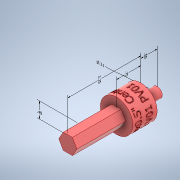
# Autodesk Inventor part: 1x8mmx1_5-inchHexShaft
Saved by Autodesk Inventor 2022.2 (Build 262287000, 287)
## iProperties
Created: 2020-11-16
Part Number: 1x8mmx1_5-inchHexShaft
Material: PC/ABS Plastic
Document SubType Name: Modeling
Designer: robst
Density: 0.357273 g/cm^3
Appearance: Smooth - Red
Author: robst
Autodesk Inventor part; units mm, degrees
ref_plane "XZ Plane" through (0, 0, 0) normal (0, 1, 0) x (-1, 0, 0)
ref_plane "XY Plane" through (0, 0, 0) normal (0, 0, 1) x (1, 0, 0)
sketch "Sketch1" plane through (0, 0, 0) normal (0, 0, 1) x (1, 0, 0)
  line L0 (7.3323, 0) -> (3.6662, -6.35)
  line L1 (3.6662, -6.35) -> (-3.6662, -6.35)
  line L2 (-3.6662, -6.35) -> (-7.3323, 0)
  line L3 (-7.3323, 0) -> (-3.6662, 6.35)
  line L4 (-3.6662, 6.35) -> (3.6662, 6.35)
  line L5 (3.6662, 6.35) -> (7.3323, 0)
  point P0 (0, 0)
  point P1 (0, 0)
  dimension "d0" = 12.7
  constraints: 12 end point, 1 coincident, 1 horizontal, 13 other
  measures "d0" distance between parallel lines of L1 L4
extrude "Hex Portion" add sketch "Sketch1" along normal mid plane 38.1
sketch "Sketch2" plane through (0, 0, -19.05) normal (0, 0, -1) x (-1, 0, 0)
  circle A0 centre (0, 0) radius 12.7
  dimension "d3" = 25.4
  constraints: 1 centre point, 1 coincident
  measures "d3" diameter of A0
extrude "Extrusion2" add sketch "Sketch2" along normal blind 19.05
thicken "Reduce Size of Hex Shaft" operation add thickness 0.1905 both sides no extend neighbours yes toward (-0.8660254, -0.5, 0) faces at (6.1103, 2.1167, -6.35) (-1.2221, 6.35, 6.35) (4.8882, -4.2333, -6.35) (-1.2221, -6.35, -6.35) (-4.8882, -4.2333, 6.35) (-6.1103, 2.1167, 6.35)
sketch "Sketch3" plane through (0, 0, -38.1) normal (0, 0, -1) x (-1, 0, 0)
  circle A0 centre (0, 0) radius 4
  dimension "d14" = 8
  constraints: 1 centre point, 1 coincident
  measures "d14" diameter of A0
extrude "Extrusion3" add sketch "Sketch3" along normal blind 12.7
ref_plane "Work Plane1" through (12.7, 0, -19.05) normal (1, 0, 0) x (0, 1, 0)
sketch "Sketch4" plane through (12.7, 0, -19.05) normal (1, 0, 0) x (0, 1, 0)
  line L0 (-12.7, 0) -> (12.7, 0) projected
  line L1 (-12.7, -19.05) -> (12.7, -19.05) projected
  line L2 (-12.7, 0) -> (-12.7, -19.05) construction
  line L3 (-12.7, -9.525) -> (12.7, -9.525) construction
  line L4 (12.7, 0) -> (12.7, -19.05) construction
  line L5 (-28.8024, -6.985) -> (-31.2807, -6.985)
  line L6 (-31.2807, -6.985) -> (-31.2807, -6.4663)
  line L7 (-31.2807, -6.4663) -> (-30.3586, -6.4663)
  line L8 (-30.3586, -6.4663) -> (-30.3586, -3.0618)
  line L9 (-30.3586, -3.0618) -> (-31.2807, -3.0618)
  line L10 (-31.2807, -3.0618) -> (-31.2807, -2.5966)
  spline S0 degree 2 poles (-31.2807, -2.5966) (-30.7579, -2.5966) (-30.2639, -2.3002) (-30.2309, -1.8885) knots 0 0 0 1 2 2 2
  line L11 (-30.2309, -1.8885) -> (-29.704, -1.8885)
  line L12 (-29.704, -1.8885) -> (-29.704, -6.4663)
  line L13 (-29.704, -6.4663) -> (-28.8024, -6.4663)
  line L14 (-28.8024, -6.4663) -> (-28.8024, -6.985)
  line L15 (-27.1064, -1.6786) -> (-27.2546, -3.6546)
  line L16 (-27.2546, -3.6546) -> (-27.7033, -3.6546)
  line L17 (-27.7033, -3.6546) -> (-27.8515, -1.6786)
  line L18 (-27.8515, -1.6786) -> (-27.1064, -1.6786)
  line L19 (-25.822, -1.6786) -> (-25.9702, -3.6546)
  line L20 (-25.9702, -3.6546) -> (-26.4189, -3.6546)
  line L21 (-26.4189, -3.6546) -> (-26.5671, -1.6786)
  line L22 (-26.5671, -1.6786) -> (-25.822, -1.6786)
  line L23 (-22.0099, -6.985) -> (-22.7962, -6.985)
  line L24 (-22.7962, -6.985) -> (-23.7224, -5.5524)
  line L25 (-23.7224, -5.5524) -> (-24.6734, -6.985)
  line L26 (-24.6734, -6.985) -> (-25.4021, -6.985)
  line L27 (-25.4021, -6.985) -> (-24.0806, -5.0954)
  line L28 (-24.0806, -5.0954) -> (-25.3897, -3.1729)
  line L29 (-25.3897, -3.1729) -> (-24.6034, -3.1729)
  line L30 (-24.6034, -3.1729) -> (-23.6813, -4.5932)
  line L31 (-23.6813, -4.5932) -> (-22.7386, -3.1729)
  line L32 (-22.7386, -3.1729) -> (-22.0099, -3.1729)
  line L33 (-22.0099, -3.1729) -> (-23.3231, -5.0543)
  line L34 (-23.3231, -5.0543) -> (-22.0099, -6.985)
  spline S1 degree 2 poles (-20.0709, -7.1003) (-20.4497, -7.1003) (-21.0713, -6.8738) (-21.2895, -6.6639) knots 0 0 0 1 2 2 2
  spline S2 degree 2 poles (-21.2895, -6.6639) (-21.5035, -6.4581) (-21.7259, -5.8982) (-21.7259, -5.5812) knots 0 0 0 1 2 2 2
  spline S3 degree 2 poles (-21.7259, -5.5812) (-21.7259, -5.1695) (-21.2854, -4.4779) (-20.8655, -4.2721) knots 0 0 0 1 2 2 2
  line L35 (-20.8655, -4.2721) -> (-20.8655, -4.2515)
  spline S4 degree 2 poles (-20.8655, -4.2515) (-21.2401, -4.0333) (-21.6024, -3.5146) (-21.6024, -3.1277) knots 0 0 0 1 2 2 2
  spline S5 degree 2 poles (-21.6024, -3.1277) (-21.6024, -2.5554) (-20.7378, -1.7897) (-20.0709, -1.7897) knots 0 0 0 1 2 2 2
  spline S6 degree 2 poles (-20.0709, -1.7897) (-19.3793, -1.7897) (-18.5436, -2.5143) (-18.5436, -3.0824) knots 0 0 0 1 2 2 2
  spline S7 degree 2 poles (-18.5436, -3.0824) (-18.5436, -3.4241) (-18.943, -4.091) (-19.3176, -4.2803) knots 0 0 0 1 2 2 2
  line L36 (-19.3176, -4.2803) -> (-19.3176, -4.3009)
  spline S8 degree 2 poles (-19.3176, -4.3009) (-18.873, -4.5068) (-18.416, -5.0996) (-18.416, -5.5689) knots 0 0 0 1 2 2 2
  spline S9 degree 2 poles (-18.416, -5.5689) (-18.416, -6.2193) (-19.3629, -7.1003) (-20.0709, -7.1003) knots 0 0 0 1 2 2 2
  spline S10 degree 2 poles (-19.1159, -5.6347) (-19.1159, -5.3219) (-19.3629, -4.9514) (-19.7128, -4.762) knots 0 0 0 1 2 2 2
  spline S11 degree 2 poles (-19.7128, -4.762) (-19.8281, -4.6961) (-20.215, -4.5438) (-20.4579, -4.445) knots 0 0 0 1 2 2 2
  spline S12 degree 2 poles (-20.4579, -4.445) (-20.7378, -4.6303) (-21.0384, -5.1819) (-21.0384, -5.5318) knots 0 0 0 1 2 2 2
  spline S13 degree 2 poles (-21.0384, -5.5318) (-21.0384, -5.9929) (-20.4826, -6.5939) (-20.0627, -6.5939) knots 0 0 0 1 2 2 2
  spline S14 degree 2 poles (-20.0627, -6.5939) (-19.6346, -6.5939) (-19.1159, -6.0793) (-19.1159, -5.6347) knots 0 0 0 1 2 2 2
  spline S15 degree 2 poles (-19.2106, -3.0906) (-19.2106, -2.7489) (-19.6675, -2.292) (-20.0751, -2.292) knots 0 0 0 1 2 2 2
  spline S16 degree 2 poles (-20.0751, -2.292) (-20.4456, -2.292) (-20.919, -2.6995) (-20.919, -3.0494) knots 0 0 0 1 2 2 2
  spline S17 degree 2 poles (-20.919, -3.0494) (-20.919, -3.3006) (-20.6761, -3.6505) (-20.4332, -3.7904) knots 0 0 0 1 2 2 2
  spline S18 degree 2 poles (-20.4332, -3.7904) (-20.3303, -3.8481) (-19.8939, -4.0498) (-19.7169, -4.1074) knots 0 0 0 1 2 2 2
  spline S19 degree 2 poles (-19.7169, -4.1074) (-19.4205, -3.881) (-19.2106, -3.3994) (-19.2106, -3.0906) knots 0 0 0 1 2 2 2
  line L37 (-13.3772, -6.985) -> (-13.3772, -4.7785)
  spline S20 degree 2 poles (-13.3772, -4.7785) (-13.3772, -4.515) (-13.4184, -4.0663) (-13.4842, -3.9428) knots 0 0 0 1 2 2 2
  spline S21 degree 2 poles (-13.4842, -3.9428) (-13.5501, -3.8069) (-13.8012, -3.6752) (-14.0194, -3.6752) knots 0 0 0 1 2 2 2
  spline S22 degree 2 poles (-14.0194, -3.6752) (-14.217, -3.6752) (-14.6698, -3.9181) (-14.9086, -4.1486) knots 0 0 0 1 2 2 2
  spline S23 degree 2 poles (-14.9086, -4.1486) (-14.9045, -4.2062) (-14.8963, -4.3668) (-14.8963, -4.4738) knots 0 0 0 1 2 2 2
  line L38 (-14.8963, -4.4738) -> (-14.8963, -6.985)
  line L39 (-14.8963, -6.985) -> (-15.5385, -6.985)
  line L40 (-15.5385, -6.985) -> (-15.5385, -4.7785)
  spline S24 degree 2 poles (-15.5385, -4.7785) (-15.5385, -4.515) (-15.5796, -4.0663) (-15.6455, -3.9428) knots 0 0 0 1 2 2 2
  spline S25 degree 2 poles (-15.6455, -3.9428) (-15.7114, -3.8069) (-15.9625, -3.6752) (-16.1807, -3.6752) knots 0 0 0 1 2 2 2
  spline S26 degree 2 poles (-16.1807, -3.6752) (-16.3865, -3.6752) (-16.8435, -3.9345) (-17.0575, -4.1362) knots 0 0 0 1 2 2 2
  line L41 (-17.0575, -4.1362) -> (-17.0575, -6.985)
  line L42 (-17.0575, -6.985) -> (-17.6997, -6.985)
  line L43 (-17.6997, -6.985) -> (-17.6997, -3.1729)
  line L44 (-17.6997, -3.1729) -> (-17.0575, -3.1729)
  line L45 (-17.0575, -3.1729) -> (-17.0575, -3.5928)
  spline S27 degree 2 poles (-17.0575, -3.5928) (-16.8064, -3.3417) (-16.3124, -3.0659) (-16.016, -3.0659) knots 0 0 0 1 2 2 2
  spline S28 degree 2 poles (-16.016, -3.0659) (-15.6784, -3.0659) (-15.1556, -3.3747) (-15.0198, -3.7246) knots 0 0 0 1 2 2 2
  spline S29 degree 2 poles (-15.0198, -3.7246) (-14.7275, -3.3994) (-14.1758, -3.0659) (-13.8547, -3.0659) knots 0 0 0 1 2 2 2
  spline S30 degree 2 poles (-13.8547, -3.0659) (-13.6077, -3.0659) (-13.2043, -3.2182) (-13.0561, -3.3911) knots 0 0 0 1 2 2 2
  spline S31 degree 2 poles (-13.0561, -3.3911) (-12.9038, -3.564) (-12.735, -4.0827) (-12.735, -4.4738) knots 0 0 0 1 2 2 2
  line L46 (-12.735, -4.4738) -> (-12.735, -6.985)
  line L47 (-12.735, -6.985) -> (-13.3772, -6.985)
  line L48 (-7.5109, -6.985) -> (-7.5109, -4.7785)
  spline S32 degree 2 poles (-7.5109, -4.7785) (-7.5109, -4.515) (-7.5521, -4.0663) (-7.6179, -3.9428) knots 0 0 0 1 2 2 2
  spline S33 degree 2 poles (-7.6179, -3.9428) (-7.6838, -3.8069) (-7.9349, -3.6752) (-8.1531, -3.6752) knots 0 0 0 1 2 2 2
  spline S34 degree 2 poles (-8.1531, -3.6752) (-8.3507, -3.6752) (-8.8035, -3.9181) (-9.0423, -4.1486) knots 0 0 0 1 2 2 2
  spline S35 degree 2 poles (-9.0423, -4.1486) (-9.0382, -4.2062) (-9.03, -4.3668) (-9.03, -4.4738) knots 0 0 0 1 2 2 2
  line L49 (-9.03, -4.4738) -> (-9.03, -6.985)
  line L50 (-9.03, -6.985) -> (-9.6722, -6.985)
  line L51 (-9.6722, -6.985) -> (-9.6722, -4.7785)
  spline S36 degree 2 poles (-9.6722, -4.7785) (-9.6722, -4.515) (-9.7133, -4.0663) (-9.7792, -3.9428) knots 0 0 0 1 2 2 2
  spline S37 degree 2 poles (-9.7792, -3.9428) (-9.8451, -3.8069) (-10.0962, -3.6752) (-10.3144, -3.6752) knots 0 0 0 1 2 2 2
  spline S38 degree 2 poles (-10.3144, -3.6752) (-10.5202, -3.6752) (-10.9772, -3.9345) (-11.1912, -4.1362) knots 0 0 0 1 2 2 2
  line L52 (-11.1912, -4.1362) -> (-11.1912, -6.985)
  line L53 (-11.1912, -6.985) -> (-11.8334, -6.985)
  line L54 (-11.8334, -6.985) -> (-11.8334, -3.1729)
  line L55 (-11.8334, -3.1729) -> (-11.1912, -3.1729)
  line L56 (-11.1912, -3.1729) -> (-11.1912, -3.5928)
  spline S39 degree 2 poles (-11.1912, -3.5928) (-10.9401, -3.3417) (-10.4461, -3.0659) (-10.1497, -3.0659) knots 0 0 0 1 2 2 2
  spline S40 degree 2 poles (-10.1497, -3.0659) (-9.8121, -3.0659) (-9.2893, -3.3747) (-9.1535, -3.7246) knots 0 0 0 1 2 2 2
  spline S41 degree 2 poles (-9.1535, -3.7246) (-8.8612, -3.3994) (-8.3095, -3.0659) (-7.9884, -3.0659) knots 0 0 0 1 2 2 2
  spline S42 degree 2 poles (-7.9884, -3.0659) (-7.7414, -3.0659) (-7.338, -3.2182) (-7.1898, -3.3911) knots 0 0 0 1 2 2 2
  spline S43 degree 2 poles (-7.1898, -3.3911) (-7.0375, -3.564) (-6.8687, -4.0827) (-6.8687, -4.4738) knots 0 0 0 1 2 2 2
  line L57 (-6.8687, -4.4738) -> (-6.8687, -6.985)
  line L58 (-6.8687, -6.985) -> (-7.5109, -6.985)
  line L59 (-3.0072, -6.985) -> (-3.7935, -6.985)
  line L60 (-3.7935, -6.985) -> (-4.7198, -5.5524)
  line L61 (-4.7198, -5.5524) -> (-5.6707, -6.985)
  line L62 (-5.6707, -6.985) -> (-6.3994, -6.985)
  line L63 (-6.3994, -6.985) -> (-5.0779, -5.0954)
  line L64 (-5.0779, -5.0954) -> (-6.3871, -3.1729)
  line L65 (-6.3871, -3.1729) -> (-5.6008, -3.1729)
  line L66 (-5.6008, -3.1729) -> (-4.6786, -4.5932)
  line L67 (-4.6786, -4.5932) -> (-3.7359, -3.1729)
  line L68 (-3.7359, -3.1729) -> (-3.0072, -3.1729)
  line L69 (-3.0072, -3.1729) -> (-4.3205, -5.0543)
  line L70 (-4.3205, -5.0543) -> (-3.0072, -6.985)
  spline S44 degree 2 poles (0.5578, -4.445) (0.5578, -5.8117) (-0.2367, -7.092) (-1.0642, -7.092) knots 0 0 0 1 2 2 2
  spline S45 degree 2 poles (-1.0642, -7.092) (-1.904, -7.092) (-2.6903, -5.787) (-2.6903, -4.4491) knots 0 0 0 1 2 2 2
  spline S46 degree 2 poles (-2.6903, -4.4491) (-2.6903, -3.0741) (-1.8957, -1.8021) (-1.0642, -1.8021) knots 0 0 0 1 2 2 2
  spline S47 degree 2 poles (-1.0642, -1.8021) (-0.2285, -1.8021) (0.5578, -3.1194) (0.5578, -4.445) knots 0 0 0 1 2 2 2
  spline S48 degree 2 poles (-0.3149, -5.9929) (-0.2161, -5.7418) (-0.1338, -4.9678) (-0.1338, -4.445) knots 0 0 0 1 2 2 2
  spline S49 degree 2 poles (-0.1338, -4.445) (-0.1338, -3.9222) (-0.2161, -3.1524) (-0.319, -2.893) knots 0 0 0 1 2 2 2
  spline S50 degree 2 poles (-0.319, -2.893) (-0.422, -2.6337) (-0.7801, -2.3661) (-1.0642, -2.3661) knots 0 0 0 1 2 2 2
  spline S51 degree 2 poles (-1.0642, -2.3661) (-1.3482, -2.3661) (-1.7146, -2.6337) (-1.8216, -2.9012) knots 0 0 0 1 2 2 2
  spline S52 degree 2 poles (-1.8216, -2.9012) (-1.9246, -3.1606) (-1.9987, -3.951) (-1.9987, -4.4491) knots 0 0 0 1 2 2 2
  spline S53 degree 2 poles (-1.9987, -4.4491) (-1.9987, -4.9843) (-1.9328, -5.7006) (-1.8258, -5.9805) knots 0 0 0 1 2 2 2
  spline S54 degree 2 poles (-1.8258, -5.9805) (-1.727, -6.244) (-1.3606, -6.528) (-1.0642, -6.528) knots 0 0 0 1 2 2 2
  spline S55 degree 2 poles (-1.0642, -6.528) (-0.7842, -6.528) (-0.4178, -6.2605) (-0.3149, -5.9929) knots 0 0 0 1 2 2 2
  line L71 (2.2992, -6.985) -> (1.4841, -6.985)
  line L72 (1.4841, -6.985) -> (1.4841, -6.0135)
  line L73 (1.4841, -6.0135) -> (2.2992, -6.0135)
  line L74 (2.2992, -6.0135) -> (2.2992, -6.985)
  spline S56 degree 2 poles (6.4035, -5.3713) (6.4035, -5.7376) (6.1689, -6.3634) (5.9548, -6.5939) knots 0 0 0 1 2 2 2
  spline S57 degree 2 poles (5.9548, -6.5939) (5.7407, -6.8244) (5.1026, -7.092) (4.7074, -7.092) knots 0 0 0 1 2 2 2
  spline S58 degree 2 poles (4.7074, -7.092) (4.3452, -7.092) (3.6371, -6.9315) (3.3777, -6.8039) knots 0 0 0 1 2 2 2
  line L75 (3.3777, -6.8039) -> (3.3777, -6.0834)
  line L76 (3.3777, -6.0834) -> (3.4271, -6.0834)
  spline S59 degree 2 poles (3.4271, -6.0834) (3.5054, -6.1411) (3.7976, -6.2893) (3.9747, -6.3551) knots 0 0 0 1 2 2 2
  spline S60 degree 2 poles (3.9747, -6.3551) (4.1764, -6.4251) (4.5098, -6.5033) (4.7198, -6.5033) knots 0 0 0 1 2 2 2
  spline S61 degree 2 poles (4.7198, -6.5033) (4.9256, -6.5033) (5.3126, -6.3551) (5.4526, -6.1946) knots 0 0 0 1 2 2 2
  spline S62 degree 2 poles (5.4526, -6.1946) (5.5802, -6.0423) (5.7119, -5.6388) (5.7119, -5.3671) knots 0 0 0 1 2 2 2
  spline S63 degree 2 poles (5.7119, -5.3671) (5.7119, -5.0954) (5.5637, -4.7496) (5.4237, -4.6344) knots 0 0 0 1 2 2 2
  spline S64 degree 2 poles (5.4237, -4.6344) (5.2797, -4.5068) (4.8515, -4.3997) (4.5922, -4.3997) knots 0 0 0 1 2 2 2
  spline S65 degree 2 poles (4.5922, -4.3997) (4.3122, -4.3997) (3.7565, -4.4862) (3.5877, -4.5232) knots 0 0 0 1 2 2 2
  line L77 (3.5877, -4.5232) -> (3.5877, -1.905)
  line L78 (3.5877, -1.905) -> (6.3747, -1.905)
  line L79 (6.3747, -1.905) -> (6.3747, -2.5019)
  line L80 (6.3747, -2.5019) -> (4.2423, -2.5019)
  line L81 (4.2423, -2.5019) -> (4.2423, -3.8563)
  spline S66 degree 2 poles (4.2423, -3.8563) (4.3658, -3.8398) (4.6045, -3.8275) (4.7033, -3.8275) knots 0 0 0 1 2 2 2
  spline S67 degree 2 poles (4.7033, -3.8275) (5.0944, -3.8275) (5.6337, -3.9551) (5.8807, -4.1445) knots 0 0 0 1 2 2 2
  spline S68 degree 2 poles (5.8807, -4.1445) (6.1318, -4.3338) (6.4035, -4.9102) (6.4035, -5.3713) knots 0 0 0 1 2 2 2
  line L82 (7.8979, -1.6786) -> (7.7497, -3.6546)
  line L83 (7.7497, -3.6546) -> (7.301, -3.6546)
  line L84 (7.301, -3.6546) -> (7.1528, -1.6786)
  line L85 (7.1528, -1.6786) -> (7.8979, -1.6786)
  line L86 (9.1823, -1.6786) -> (9.0341, -3.6546)
  line L87 (9.0341, -3.6546) -> (8.5854, -3.6546)
  line L88 (8.5854, -3.6546) -> (8.4372, -1.6786)
  line L89 (8.4372, -1.6786) -> (9.1823, -1.6786)
  spline S69 degree 2 poles (14.2499, -7.0756) (13.7559, -7.0756) (12.9202, -6.7421) (12.6156, -6.4087) knots 0 0 0 1 2 2 2
  spline S70 degree 2 poles (12.6156, -6.4087) (12.311, -6.0793) (11.9775, -5.0913) (11.9775, -4.4491) knots 0 0 0 1 2 2 2
  spline S71 degree 2 poles (11.9775, -4.4491) (11.9775, -3.811) (12.3027, -2.8642) (12.6115, -2.5143) knots 0 0 0 1 2 2 2
  spline S72 degree 2 poles (12.6115, -2.5143) (12.9161, -2.1726) (13.7477, -1.8144) (14.2623, -1.8144) knots 0 0 0 1 2 2 2
  spline S73 degree 2 poles (14.2623, -1.8144) (14.5175, -1.8144) (14.9662, -1.8885) (15.1556, -1.9462) knots 0 0 0 1 2 2 2
  spline S74 degree 2 poles (15.1556, -1.9462) (15.3203, -1.9997) (15.662, -2.152) (15.8307, -2.2426) knots 0 0 0 1 2 2 2
  line L90 (15.8307, -2.2426) -> (15.8307, -3.0577)
  line L91 (15.8307, -3.0577) -> (15.7772, -3.0577)
  spline S75 degree 2 poles (15.7772, -3.0577) (15.6867, -2.9753) (15.4067, -2.7448) (15.205, -2.6337) knots 0 0 0 1 2 2 2
  spline S76 degree 2 poles (15.205, -2.6337) (15.0115, -2.5266) (14.5546, -2.3908) (14.2582, -2.3908) knots 0 0 0 1 2 2 2
  spline S77 degree 2 poles (14.2582, -2.3908) (13.9329, -2.3908) (13.3525, -2.6584) (13.1343, -2.9136) knots 0 0 0 1 2 2 2
  spline S78 degree 2 poles (13.1343, -2.9136) (12.9202, -3.1729) (12.6815, -3.9592) (12.6815, -4.4491) knots 0 0 0 1 2 2 2
  spline S79 degree 2 poles (12.6815, -4.4491) (12.6815, -4.9719) (12.9326, -5.7253) (13.1508, -5.9846) knots 0 0 0 1 2 2 2
  spline S80 degree 2 poles (13.1508, -5.9846) (13.3648, -6.2358) (13.9371, -6.491) (14.2582, -6.491) knots 0 0 0 1 2 2 2
  spline S81 degree 2 poles (14.2582, -6.491) (14.5505, -6.491) (15.0486, -6.3469) (15.2421, -6.2399) knots 0 0 0 1 2 2 2
  spline S82 degree 2 poles (15.2421, -6.2399) (15.4273, -6.1328) (15.7031, -5.9105) (15.7813, -5.8323) knots 0 0 0 1 2 2 2
  line L92 (15.7813, -5.8323) -> (15.8307, -5.8323)
  line L93 (15.8307, -5.8323) -> (15.8307, -6.6392)
  spline S83 degree 2 poles (15.8307, -6.6392) (15.662, -6.7174) (15.3656, -6.8615) (15.1556, -6.9274) knots 0 0 0 1 2 2 2
  spline S84 degree 2 poles (15.1556, -6.9274) (14.9333, -7.0015) (14.5546, -7.0756) (14.2499, -7.0756) knots 0 0 0 1 2 2 2
  spline S85 degree 2 poles (18.0661, -7.0715) (17.1522, -7.0715) (16.1477, -6.0464) (16.1477, -5.0996) knots 0 0 0 1 2 2 2
  spline S86 degree 2 poles (16.1477, -5.0996) (16.1477, -4.1692) (17.1234, -3.0659) (17.9097, -3.0659) knots 0 0 0 1 2 2 2
  spline S87 degree 2 poles (17.9097, -3.0659) (18.2637, -3.0659) (18.8112, -3.2717) (19.0129, -3.4899) knots 0 0 0 1 2 2 2
  spline S88 degree 2 poles (19.0129, -3.4899) (19.2188, -3.7081) (19.437, -4.338) (19.437, -4.7949) knots 0 0 0 1 2 2 2
  line L94 (19.437, -4.7949) -> (19.437, -5.1448)
  line L95 (19.437, -5.1448) -> (16.7982, -5.1448)
  spline S89 degree 2 poles (16.7982, -5.1448) (16.7982, -5.8076) (17.4651, -6.5116) (18.0579, -6.5116) knots 0 0 0 1 2 2 2
  spline S90 degree 2 poles (18.0579, -6.5116) (18.2678, -6.5116) (18.6754, -6.4169) (18.84, -6.3428) knots 0 0 0 1 2 2 2
  spline S91 degree 2 poles (18.84, -6.3428) (19.0129, -6.2605) (19.2517, -6.1164) (19.3299, -6.0505) knots 0 0 0 1 2 2 2
  line L96 (19.3299, -6.0505) -> (19.367, -6.0505)
  line L97 (19.367, -6.0505) -> (19.367, -6.7503)
  spline S92 degree 2 poles (19.367, -6.7503) (19.2558, -6.7956) (18.9183, -6.9274) (18.7865, -6.9644) knots 0 0 0 1 2 2 2
  spline S93 degree 2 poles (18.7865, -6.9644) (18.6013, -7.0179) (18.2966, -7.0715) (18.0661, -7.0715) knots 0 0 0 1 2 2 2
  spline S94 degree 2 poles (18.8112, -4.655) (18.803, -4.3956) (18.696, -4.0169) (18.593, -3.8892) knots 0 0 0 1 2 2 2
  spline S95 degree 2 poles (18.593, -3.8892) (18.4819, -3.7452) (18.132, -3.5928) (17.8726, -3.5928) knots 0 0 0 1 2 2 2
  spline S96 degree 2 poles (17.8726, -3.5928) (17.6174, -3.5928) (17.2592, -3.7452) (17.111, -3.8934) knots 0 0 0 1 2 2 2
  spline S97 degree 2 poles (17.111, -3.8934) (16.967, -4.0457) (16.8188, -4.4121) (16.7982, -4.655) knots 0 0 0 1 2 2 2
  line L98 (16.7982, -4.655) -> (18.8112, -4.655)
  line L99 (23.0802, -6.985) -> (22.438, -6.985)
  line L100 (22.438, -6.985) -> (22.438, -4.8114)
  spline S98 degree 2 poles (22.438, -4.8114) (22.438, -4.5479) (22.3886, -4.0951) (22.3145, -3.9592) knots 0 0 0 1 2 2 2
  spline S99 degree 2 poles (22.3145, -3.9592) (22.2363, -3.8151) (21.9564, -3.6752) (21.7176, -3.6752) knots 0 0 0 1 2 2 2
  spline S100 degree 2 poles (21.7176, -3.6752) (21.4788, -3.6752) (20.9725, -3.9304) (20.7296, -4.1362) knots 0 0 0 1 2 2 2
  line L101 (20.7296, -4.1362) -> (20.7296, -6.985)
  line L102 (20.7296, -6.985) -> (20.0874, -6.985)
  line L103 (20.0874, -6.985) -> (20.0874, -3.1729)
  line L104 (20.0874, -3.1729) -> (20.7296, -3.1729)
  line L105 (20.7296, -3.1729) -> (20.7296, -3.597)
  spline S101 degree 2 poles (20.7296, -3.597) (21.0178, -3.3376) (21.5735, -3.0659) (21.8864, -3.0659) knots 0 0 0 1 2 2 2
  spline S102 degree 2 poles (21.8864, -3.0659) (22.4463, -3.0659) (23.0802, -3.8069) (23.0802, -4.5109) knots 0 0 0 1 2 2 2
  line L106 (23.0802, -4.5109) -> (23.0802, -6.985)
  spline S103 degree 2 poles (25.1345, -7.0591) (24.6117, -7.0591) (24.023, -6.4622) (24.023, -5.8159) knots 0 0 0 1 2 2 2
  line L107 (24.023, -5.8159) -> (24.023, -3.704)
  line L108 (24.023, -3.704) -> (23.5907, -3.704)
  line L109 (23.5907, -3.704) -> (23.5907, -3.1729)
  line L110 (23.5907, -3.1729) -> (24.023, -3.1729)
  line L111 (24.023, -3.1729) -> (24.023, -2.0779)
  line L112 (24.023, -2.0779) -> (24.6652, -2.0779)
  line L113 (24.6652, -2.0779) -> (24.6652, -3.1729)
  line L114 (24.6652, -3.1729) -> (25.8467, -3.1729)
  line L115 (25.8467, -3.1729) -> (25.8467, -3.704)
  line L116 (25.8467, -3.704) -> (24.6652, -3.704)
  line L117 (24.6652, -3.704) -> (24.6652, -5.5195)
  spline S104 degree 2 poles (24.6652, -5.5195) (24.6652, -5.8076) (24.6858, -6.1246) (24.7557, -6.2605) knots 0 0 0 1 2 2 2
  spline S105 degree 2 poles (24.7557, -6.2605) (24.8134, -6.3798) (25.0727, -6.4992) (25.295, -6.4992) knots 0 0 0 1 2 2 2
  spline S106 degree 2 poles (25.295, -6.4992) (25.4515, -6.4992) (25.7437, -6.4045) (25.8096, -6.3757) knots 0 0 0 1 2 2 2
  line L118 (25.8096, -6.3757) -> (25.8467, -6.3757)
  line L119 (25.8467, -6.3757) -> (25.8467, -6.9521)
  spline S107 degree 2 poles (25.8467, -6.9521) (25.6655, -7.0015) (25.295, -7.0591) (25.1345, -7.0591) knots 0 0 0 1 2 2 2
  spline S108 degree 2 poles (27.975, -7.0715) (27.0611, -7.0715) (26.0566, -6.0464) (26.0566, -5.0996) knots 0 0 0 1 2 2 2
  spline S109 degree 2 poles (26.0566, -5.0996) (26.0566, -4.1692) (27.0323, -3.0659) (27.8186, -3.0659) knots 0 0 0 1 2 2 2
  spline S110 degree 2 poles (27.8186, -3.0659) (28.1726, -3.0659) (28.7201, -3.2717) (28.9218, -3.4899) knots 0 0 0 1 2 2 2
  spline S111 degree 2 poles (28.9218, -3.4899) (29.1277, -3.7081) (29.3459, -4.338) (29.3459, -4.7949) knots 0 0 0 1 2 2 2
  line L120 (29.3459, -4.7949) -> (29.3459, -5.1448)
  line L121 (29.3459, -5.1448) -> (26.7071, -5.1448)
  spline S112 degree 2 poles (26.7071, -5.1448) (26.7071, -5.8076) (27.374, -6.5116) (27.9668, -6.5116) knots 0 0 0 1 2 2 2
  spline S113 degree 2 poles (27.9668, -6.5116) (28.1767, -6.5116) (28.5843, -6.4169) (28.7489, -6.3428) knots 0 0 0 1 2 2 2
  spline S114 degree 2 poles (28.7489, -6.3428) (28.9218, -6.2605) (29.1606, -6.1164) (29.2388, -6.0505) knots 0 0 0 1 2 2 2
  line L122 (29.2388, -6.0505) -> (29.2759, -6.0505)
  line L123 (29.2759, -6.0505) -> (29.2759, -6.7503)
  spline S115 degree 2 poles (29.2759, -6.7503) (29.1647, -6.7956) (28.8271, -6.9274) (28.6954, -6.9644) knots 0 0 0 1 2 2 2
  spline S116 degree 2 poles (28.6954, -6.9644) (28.5102, -7.0179) (28.2055, -7.0715) (27.975, -7.0715) knots 0 0 0 1 2 2 2
  spline S117 degree 2 poles (28.7201, -4.655) (28.7119, -4.3956) (28.6048, -4.0169) (28.5019, -3.8892) knots 0 0 0 1 2 2 2
  spline S118 degree 2 poles (28.5019, -3.8892) (28.3908, -3.7452) (28.0409, -3.5928) (27.7815, -3.5928) knots 0 0 0 1 2 2 2
  spline S119 degree 2 poles (27.7815, -3.5928) (27.5263, -3.5928) (27.1681, -3.7452) (27.0199, -3.8934) knots 0 0 0 1 2 2 2
  spline S120 degree 2 poles (27.0199, -3.8934) (26.8758, -4.0457) (26.7276, -4.4121) (26.7071, -4.655) knots 0 0 0 1 2 2 2
  line L124 (26.7071, -4.655) -> (28.7201, -4.655)
  line L125 (32.0176, -3.8604) -> (31.9847, -3.8604)
  spline S121 degree 2 poles (31.9847, -3.8604) (31.9106, -3.8398) (31.75, -3.8316) (31.6388, -3.8316) knots 0 0 0 1 2 2 2
  spline S122 degree 2 poles (31.6388, -3.8316) (31.3795, -3.8316) (30.869, -4.058) (30.6385, -4.2803) knots 0 0 0 1 2 2 2
  line L126 (30.6385, -4.2803) -> (30.6385, -6.985)
  line L127 (30.6385, -6.985) -> (29.9963, -6.985)
  line L128 (29.9963, -6.985) -> (29.9963, -3.1729)
  line L129 (29.9963, -3.1729) -> (30.6385, -3.1729)
  line L130 (30.6385, -3.1729) -> (30.6385, -3.741)
  spline S123 degree 2 poles (30.6385, -3.741) (30.9884, -3.4282) (31.5112, -3.1729) (31.7582, -3.1729) knots 0 0 0 1 2 2 2
  spline S124 degree 2 poles (31.7582, -3.1729) (31.857, -3.1729) (31.9558, -3.1812) (32.0176, -3.1935) knots 0 0 0 1 2 2 2
  line L131 (32.0176, -3.1935) -> (32.0176, -3.8604)
  spline S125 degree 2 poles (-21.979, -15.6168) (-22.5307, -15.6168) (-23.3046, -15.3863) (-23.6463, -15.2216) knots 0 0 0 1 2 2 2
  line L132 (-23.6463, -15.2216) -> (-23.6463, -14.3735)
  line L133 (-23.6463, -14.3735) -> (-23.5969, -14.3735)
  spline S126 degree 2 poles (-23.5969, -14.3735) (-23.2634, -14.6864) (-22.4195, -15.0322) (-22.0284, -15.0322) knots 0 0 0 1 2 2 2
  spline S127 degree 2 poles (-22.0284, -15.0322) (-21.4686, -15.0322) (-20.8963, -14.567) (-20.8963, -14.1842) knots 0 0 0 1 2 2 2
  spline S128 degree 2 poles (-20.8963, -14.1842) (-20.8963, -13.8795) (-21.1969, -13.5008) (-21.5221, -13.4061) knots 0 0 0 1 2 2 2
  spline S129 degree 2 poles (-21.5221, -13.4061) (-21.7567, -13.3403) (-22.1478, -13.2497) (-22.4401, -13.1756) knots 0 0 0 1 2 2 2
  spline S130 degree 2 poles (-22.4401, -13.1756) (-22.7036, -13.1056) (-23.1194, -12.8957) (-23.2799, -12.7269) knots 0 0 0 1 2 2 2
  spline S131 degree 2 poles (-23.2799, -12.7269) (-23.4363, -12.5581) (-23.6092, -12.1053) (-23.6092, -11.8088) knots 0 0 0 1 2 2 2
  spline S132 degree 2 poles (-23.6092, -11.8088) (-23.6092, -11.1913) (-22.6459, -10.3557) (-21.9008, -10.3557) knots 0 0 0 1 2 2 2
  spline S133 degree 2 poles (-21.9008, -10.3557) (-21.4727, -10.3557) (-20.7152, -10.5244) (-20.39, -10.685) knots 0 0 0 1 2 2 2
  line L134 (-20.39, -10.685) -> (-20.39, -11.4919)
  line L135 (-20.39, -11.4919) -> (-20.4394, -11.4919)
  spline S134 degree 2 poles (-20.4394, -11.4919) (-20.6823, -11.2696) (-21.4397, -10.9402) (-21.8555, -10.9402) knots 0 0 0 1 2 2 2
  spline S135 degree 2 poles (-21.8555, -10.9402) (-22.3248, -10.9402) (-22.9053, -11.3807) (-22.9053, -11.7389) knots 0 0 0 1 2 2 2
  spline S136 degree 2 poles (-22.9053, -11.7389) (-22.9053, -12.06) (-22.5636, -12.4428) (-22.2425, -12.5293) knots 0 0 0 1 2 2 2
  spline S137 degree 2 poles (-22.2425, -12.5293) (-22.0284, -12.5869) (-21.4068, -12.7351) (-21.201, -12.7969) knots 0 0 0 1 2 2 2
  spline S138 degree 2 poles (-21.201, -12.7969) (-20.6782, -12.9574) (-20.1924, -13.6037) (-20.1924, -14.0771) knots 0 0 0 1 2 2 2
  spline S139 degree 2 poles (-20.1924, -14.0771) (-20.1924, -14.3777) (-20.4353, -14.954) (-20.6535, -15.1557) knots 0 0 0 1 2 2 2
  spline S140 degree 2 poles (-20.6535, -15.1557) (-20.8963, -15.378) (-21.5138, -15.6168) (-21.979, -15.6168) knots 0 0 0 1 2 2 2
  line L136 (-16.5615, -15.5262) -> (-17.2037, -15.5262)
  line L137 (-17.2037, -15.5262) -> (-17.2037, -13.3526)
  spline S141 degree 2 poles (-17.2037, -13.3526) (-17.2037, -13.0891) (-17.2531, -12.6363) (-17.3272, -12.5005) knots 0 0 0 1 2 2 2
  spline S142 degree 2 poles (-17.3272, -12.5005) (-17.4054, -12.3564) (-17.6853, -12.2164) (-17.9241, -12.2164) knots 0 0 0 1 2 2 2
  spline S143 degree 2 poles (-17.9241, -12.2164) (-18.1629, -12.2164) (-18.6692, -12.4716) (-18.9121, -12.6775) knots 0 0 0 1 2 2 2
  line L138 (-18.9121, -12.6775) -> (-18.9121, -15.5262)
  line L139 (-18.9121, -15.5262) -> (-19.5543, -15.5262)
  line L140 (-19.5543, -15.5262) -> (-19.5543, -10.2198)
  line L141 (-19.5543, -10.2198) -> (-18.9121, -10.2198)
  line L142 (-18.9121, -10.2198) -> (-18.9121, -12.1382)
  spline S144 degree 2 poles (-18.9121, -12.1382) (-18.6239, -11.8788) (-18.0682, -11.6071) (-17.7553, -11.6071) knots 0 0 0 1 2 2 2
  spline S145 degree 2 poles (-17.7553, -11.6071) (-17.1954, -11.6071) (-16.5615, -12.3481) (-16.5615, -13.0521) knots 0 0 0 1 2 2 2
  line L143 (-16.5615, -13.0521) -> (-16.5615, -15.5262)
  spline S146 degree 2 poles (-13.5357, -15.1228) (-13.6139, -15.1804) (-13.8774, -15.3863) (-14.0009, -15.448) knots 0 0 0 1 2 2 2
  spline S147 degree 2 poles (-14.0009, -15.448) (-14.1697, -15.5386) (-14.4866, -15.6333) (-14.7748, -15.6333) knots 0 0 0 1 2 2 2
  spline S148 degree 2 poles (-14.7748, -15.6333) (-15.0095, -15.6333) (-15.4335, -15.4562) (-15.594, -15.2957) knots 0 0 0 1 2 2 2
  spline S149 degree 2 poles (-15.594, -15.2957) (-15.7464, -15.1393) (-15.9316, -14.6782) (-15.9316, -14.4229) knots 0 0 0 1 2 2 2
  spline S150 degree 2 poles (-15.9316, -14.4229) (-15.9316, -14.0277) (-15.5982, -13.4679) (-15.2359, -13.3073) knots 0 0 0 1 2 2 2
  spline S151 degree 2 poles (-15.2359, -13.3073) (-14.9148, -13.1591) (-14.042, -13.048) (-13.5357, -13.0192) knots 0 0 0 1 2 2 2
  line L144 (-13.5357, -13.0192) -> (-13.5357, -12.8957)
  spline S152 degree 2 poles (-13.5357, -12.8957) (-13.5357, -12.6734) (-13.6715, -12.3975) (-13.795, -12.3193) knots 0 0 0 1 2 2 2
  spline S153 degree 2 poles (-13.795, -12.3193) (-13.9185, -12.2411) (-14.2726, -12.1917) (-14.4619, -12.1917) knots 0 0 0 1 2 2 2
  spline S154 degree 2 poles (-14.4619, -12.1917) (-14.6842, -12.1917) (-15.2853, -12.3234) (-15.5858, -12.4511) knots 0 0 0 1 2 2 2
  line L145 (-15.5858, -12.4511) -> (-15.6229, -12.4511)
  line L146 (-15.6229, -12.4511) -> (-15.6229, -11.7965)
  spline S155 degree 2 poles (-15.6229, -11.7965) (-15.4458, -11.7471) (-14.783, -11.6236) (-14.4578, -11.6236) knots 0 0 0 1 2 2 2
  spline S156 degree 2 poles (-14.4578, -11.6236) (-14.0626, -11.6236) (-13.5233, -11.7471) (-13.3093, -11.9076) knots 0 0 0 1 2 2 2
  spline S157 degree 2 poles (-13.3093, -11.9076) (-13.0993, -12.0641) (-12.8935, -12.5622) (-12.8935, -12.9204) knots 0 0 0 1 2 2 2
  line L147 (-12.8935, -12.9204) -> (-12.8935, -15.5262)
  line L148 (-12.8935, -15.5262) -> (-13.5357, -15.5262)
  line L149 (-13.5357, -15.5262) -> (-13.5357, -15.1228)
  line L150 (-13.5357, -14.5876) -> (-13.5357, -13.5296)
  spline S158 degree 2 poles (-13.5357, -13.5296) (-13.7662, -13.5502) (-14.4619, -13.6202) (-14.6801, -13.6861) knots 0 0 0 1 2 2 2
  spline S159 degree 2 poles (-14.6801, -13.6861) (-14.9354, -13.7643) (-15.2688, -14.0895) (-15.2688, -14.3777) knots 0 0 0 1 2 2 2
  spline S160 degree 2 poles (-15.2688, -14.3777) (-15.2688, -14.707) (-14.8983, -15.0405) (-14.5443, -15.0405) knots 0 0 0 1 2 2 2
  spline S161 degree 2 poles (-14.5443, -15.0405) (-14.2438, -15.0405) (-13.7498, -14.7811) (-13.5357, -14.5876) knots 0 0 0 1 2 2 2
  line L151 (-9.9871, -10.8373) -> (-10.02, -10.8373)
  spline S162 degree 2 poles (-10.02, -10.8373) (-10.1065, -10.8044) (-10.4276, -10.7467) (-10.5552, -10.7467) knots 0 0 0 1 2 2 2
  spline S163 degree 2 poles (-10.5552, -10.7467) (-10.9586, -10.7467) (-11.3044, -11.109) (-11.3044, -11.5865) knots 0 0 0 1 2 2 2
  line L152 (-11.3044, -11.5865) -> (-11.3044, -11.7142)
  line L153 (-11.3044, -11.7142) -> (-10.2423, -11.7142)
  line L154 (-10.2423, -11.7142) -> (-10.2423, -12.2452)
  line L155 (-10.2423, -12.2452) -> (-11.2839, -12.2452)
  line L156 (-11.2839, -12.2452) -> (-11.2839, -15.5262)
  line L157 (-11.2839, -15.5262) -> (-11.9261, -15.5262)
  line L158 (-11.9261, -15.5262) -> (-11.9261, -12.2452)
  line L159 (-11.9261, -12.2452) -> (-12.3583, -12.2452)
  line L160 (-12.3583, -12.2452) -> (-12.3583, -11.7142)
  line L161 (-12.3583, -11.7142) -> (-11.9261, -11.7142)
  line L162 (-11.9261, -11.7142) -> (-11.9261, -11.5865)
  spline S164 degree 2 poles (-11.9261, -11.5865) (-11.9261, -10.9032) (-11.2633, -10.1869) (-10.6458, -10.1869) knots 0 0 0 1 2 2 2
  spline S165 degree 2 poles (-10.6458, -10.1869) (-10.4688, -10.1869) (-10.1271, -10.2239) (-9.9871, -10.2486) knots 0 0 0 1 2 2 2
  line L163 (-9.9871, -10.2486) -> (-9.9871, -10.8373)
  spline S166 degree 2 poles (-8.468, -15.6003) (-8.9909, -15.6003) (-9.5795, -15.0034) (-9.5795, -14.3571) knots 0 0 0 1 2 2 2
  line L164 (-9.5795, -14.3571) -> (-9.5795, -12.2452)
  line L165 (-9.5795, -12.2452) -> (-10.0118, -12.2452)
  line L166 (-10.0118, -12.2452) -> (-10.0118, -11.7142)
  line L167 (-10.0118, -11.7142) -> (-9.5795, -11.7142)
  line L168 (-9.5795, -11.7142) -> (-9.5795, -10.6191)
  line L169 (-9.5795, -10.6191) -> (-8.9373, -10.6191)
  line L170 (-8.9373, -10.6191) -> (-8.9373, -11.7142)
  line L171 (-8.9373, -11.7142) -> (-7.7559, -11.7142)
  line L172 (-7.7559, -11.7142) -> (-7.7559, -12.2452)
  line L173 (-7.7559, -12.2452) -> (-8.9373, -12.2452)
  line L174 (-8.9373, -12.2452) -> (-8.9373, -14.0607)
  spline S167 degree 2 poles (-8.9373, -14.0607) (-8.9373, -14.3488) (-8.9168, -14.6658) (-8.8468, -14.8017) knots 0 0 0 1 2 2 2
  spline S168 degree 2 poles (-8.8468, -14.8017) (-8.7891, -14.9211) (-8.5298, -15.0405) (-8.3075, -15.0405) knots 0 0 0 1 2 2 2
  spline S169 degree 2 poles (-8.3075, -15.0405) (-8.1511, -15.0405) (-7.8588, -14.9458) (-7.7929, -14.917) knots 0 0 0 1 2 2 2
  line L175 (-7.7929, -14.917) -> (-7.7559, -14.917)
  line L176 (-7.7559, -14.917) -> (-7.7559, -15.4933)
  spline S170 degree 2 poles (-7.7559, -15.4933) (-7.937, -15.5427) (-8.3075, -15.6003) (-8.468, -15.6003) knots 0 0 0 1 2 2 2
  line L177 (-1.3667, -10.4462) -> (-3.1163, -15.5262)
  line L178 (-3.1163, -15.5262) -> (-3.845, -15.5262)
  line L179 (-3.845, -15.5262) -> (-5.5946, -10.4462)
  line L180 (-5.5946, -10.4462) -> (-4.87, -10.4462)
  line L181 (-4.87, -10.4462) -> (-3.4621, -14.6658)
  line L182 (-3.4621, -14.6658) -> (-2.0542, -10.4462)
  line L183 (-2.0542, -10.4462) -> (-1.3667, -10.4462)
  spline S171 degree 2 poles (2.1942, -12.9862) (2.1942, -14.353) (1.3997, -15.6333) (0.5722, -15.6333) knots 0 0 0 1 2 2 2
  spline S172 degree 2 poles (0.5722, -15.6333) (-0.2676, -15.6333) (-1.0539, -14.3283) (-1.0539, -12.9903) knots 0 0 0 1 2 2 2
  spline S173 degree 2 poles (-1.0539, -12.9903) (-1.0539, -11.6154) (-0.2594, -10.3433) (0.5722, -10.3433) knots 0 0 0 1 2 2 2
  spline S174 degree 2 poles (0.5722, -10.3433) (1.4079, -10.3433) (2.1942, -11.6606) (2.1942, -12.9862) knots 0 0 0 1 2 2 2
  spline S175 degree 2 poles (1.3215, -14.5341) (1.4203, -14.283) (1.5026, -13.509) (1.5026, -12.9862) knots 0 0 0 1 2 2 2
  spline S176 degree 2 poles (1.5026, -12.9862) (1.5026, -12.4634) (1.4203, -11.6936) (1.3173, -11.4342) knots 0 0 0 1 2 2 2
  spline S177 degree 2 poles (1.3173, -11.4342) (1.2144, -11.1749) (0.8563, -10.9073) (0.5722, -10.9073) knots 0 0 0 1 2 2 2
  spline S178 degree 2 poles (0.5722, -10.9073) (0.2882, -10.9073) (-0.0782, -11.1749) (-0.1853, -11.4425) knots 0 0 0 1 2 2 2
  spline S179 degree 2 poles (-0.1853, -11.4425) (-0.2882, -11.7018) (-0.3623, -12.4922) (-0.3623, -12.9903) knots 0 0 0 1 2 2 2
  spline S180 degree 2 poles (-0.3623, -12.9903) (-0.3623, -13.5255) (-0.2964, -14.2418) (-0.1894, -14.5217) knots 0 0 0 1 2 2 2
  spline S181 degree 2 poles (-0.1894, -14.5217) (-0.0906, -14.7852) (0.2758, -15.0693) (0.5722, -15.0693) knots 0 0 0 1 2 2 2
  spline S182 degree 2 poles (0.5722, -15.0693) (0.8522, -15.0693) (1.2185, -14.8017) (1.3215, -14.5341) knots 0 0 0 1 2 2 2
  line L184 (5.7222, -15.5262) -> (3.244, -15.5262)
  line L185 (3.244, -15.5262) -> (3.244, -15.0075)
  line L186 (3.244, -15.0075) -> (4.1661, -15.0075)
  line L187 (4.1661, -15.0075) -> (4.1661, -11.603)
  line L188 (4.1661, -11.603) -> (3.244, -11.603)
  line L189 (3.244, -11.603) -> (3.244, -11.1378)
  spline S183 degree 2 poles (3.244, -11.1378) (3.7668, -11.1378) (4.2608, -10.8414) (4.2937, -10.4298) knots 0 0 0 1 2 2 2
  line L190 (4.2937, -10.4298) -> (4.8206, -10.4298)
  line L191 (4.8206, -10.4298) -> (4.8206, -15.0075)
  line L192 (4.8206, -15.0075) -> (5.7222, -15.0075)
  line L193 (5.7222, -15.0075) -> (5.7222, -15.5262)
  spline S184 degree 2 poles (12.1936, -11.9776) (12.1936, -12.307) (11.959, -12.8998) (11.749, -13.1056) knots 0 0 0 1 2 2 2
  spline S185 degree 2 poles (11.749, -13.1056) (11.4856, -13.365) (10.7734, -13.6325) (10.23, -13.6325) knots 0 0 0 1 2 2 2
  line L194 (10.23, -13.6325) -> (9.6578, -13.6325)
  line L195 (9.6578, -13.6325) -> (9.6578, -15.5262)
  line L196 (9.6578, -15.5262) -> (8.9826, -15.5262)
  line L197 (8.9826, -15.5262) -> (8.9826, -10.4462)
  line L198 (8.9826, -10.4462) -> (10.2588, -10.4462)
  spline S186 degree 2 poles (10.2588, -10.4462) (10.7116, -10.4462) (11.3456, -10.5944) (11.5885, -10.7632) knots 0 0 0 1 2 2 2
  spline S187 degree 2 poles (11.5885, -10.7632) (11.8725, -10.9567) (12.1936, -11.5536) (12.1936, -11.9776) knots 0 0 0 1 2 2 2
  spline S188 degree 2 poles (11.4897, -11.9982) (11.4897, -11.7347) (11.3086, -11.3478) (11.1233, -11.2243) knots 0 0 0 1 2 2 2
  spline S189 degree 2 poles (11.1233, -11.2243) (10.9628, -11.1172) (10.5346, -11.0308) (10.2176, -11.0308) knots 0 0 0 1 2 2 2
  line L199 (10.2176, -11.0308) -> (9.6578, -11.0308)
  line L200 (9.6578, -11.0308) -> (9.6578, -13.0562)
  line L201 (9.6578, -13.0562) -> (10.1188, -13.0562)
  spline S190 degree 2 poles (10.1188, -13.0562) (10.5305, -13.0562) (11.0369, -12.9245) (11.2015, -12.7516) knots 0 0 0 1 2 2 2
  spline S191 degree 2 poles (11.2015, -12.7516) (11.3538, -12.5993) (11.4897, -12.2411) (11.4897, -11.9982) knots 0 0 0 1 2 2 2
  line L202 (16.5203, -10.4462) -> (14.7707, -15.5262)
  line L203 (14.7707, -15.5262) -> (14.042, -15.5262)
  line L204 (14.042, -15.5262) -> (12.2924, -10.4462)
  line L205 (12.2924, -10.4462) -> (13.017, -10.4462)
  line L206 (13.017, -10.4462) -> (14.4249, -14.6658)
  line L207 (14.4249, -14.6658) -> (15.8328, -10.4462)
  line L208 (15.8328, -10.4462) -> (16.5203, -10.4462)
  spline S192 degree 2 poles (20.0812, -12.9862) (20.0812, -14.353) (19.2867, -15.6333) (18.4593, -15.6333) knots 0 0 0 1 2 2 2
  spline S193 degree 2 poles (18.4593, -15.6333) (17.6194, -15.6333) (16.8332, -14.3283) (16.8332, -12.9903) knots 0 0 0 1 2 2 2
  spline S194 degree 2 poles (16.8332, -12.9903) (16.8332, -11.6154) (17.6277, -10.3433) (18.4593, -10.3433) knots 0 0 0 1 2 2 2
  spline S195 degree 2 poles (18.4593, -10.3433) (19.2949, -10.3433) (20.0812, -11.6606) (20.0812, -12.9862) knots 0 0 0 1 2 2 2
  spline S196 degree 2 poles (19.2085, -14.5341) (19.3073, -14.283) (19.3896, -13.509) (19.3896, -12.9862) knots 0 0 0 1 2 2 2
  spline S197 degree 2 poles (19.3896, -12.9862) (19.3896, -12.4634) (19.3073, -11.6936) (19.2044, -11.4342) knots 0 0 0 1 2 2 2
  spline S198 degree 2 poles (19.2044, -11.4342) (19.1015, -11.1749) (18.7433, -10.9073) (18.4593, -10.9073) knots 0 0 0 1 2 2 2
  spline S199 degree 2 poles (18.4593, -10.9073) (18.1752, -10.9073) (17.8088, -11.1749) (17.7018, -11.4425) knots 0 0 0 1 2 2 2
  spline S200 degree 2 poles (17.7018, -11.4425) (17.5989, -11.7018) (17.5248, -12.4922) (17.5248, -12.9903) knots 0 0 0 1 2 2 2
  spline S201 degree 2 poles (17.5248, -12.9903) (17.5248, -13.5255) (17.5906, -14.2418) (17.6977, -14.5217) knots 0 0 0 1 2 2 2
  spline S202 degree 2 poles (17.6977, -14.5217) (17.7965, -14.7852) (18.1629, -15.0693) (18.4593, -15.0693) knots 0 0 0 1 2 2 2
  spline S203 degree 2 poles (18.4593, -15.0693) (18.7392, -15.0693) (19.1056, -14.8017) (19.2085, -14.5341) knots 0 0 0 1 2 2 2
  line L209 (23.6092, -15.5262) -> (21.131, -15.5262)
  line L210 (21.131, -15.5262) -> (21.131, -15.0075)
  line L211 (21.131, -15.0075) -> (22.0531, -15.0075)
  line L212 (22.0531, -15.0075) -> (22.0531, -11.603)
  line L213 (22.0531, -11.603) -> (21.131, -11.603)
  line L214 (21.131, -11.603) -> (21.131, -11.1378)
  spline S204 degree 2 poles (21.131, -11.1378) (21.6538, -11.1378) (22.1478, -10.8414) (22.1807, -10.4298) knots 0 0 0 1 2 2 2
  line L215 (22.1807, -10.4298) -> (22.7077, -10.4298)
  line L216 (22.7077, -10.4298) -> (22.7077, -15.0075)
  line L217 (22.7077, -15.0075) -> (23.6092, -15.0075)
  line L218 (23.6092, -15.0075) -> (23.6092, -15.5262)
  point P0 (0, 19.05)
  constraints: 2 end point, 2 midpoint, 1 horizontal
emboss "Emboss1" sketch "Sketch4" operation cut depth 2.54 direction (-1, 0, 0) wrap yes faces at (-12.6588, 1.0219, -25.4)
equation "\"d0\" = hexSize"
equation "\"d1\" = length"
equation "\"d6\" = printOffset"
equation "\"hexSize\" = 12.7"
equation "\"length\" = 38.1"
equation "\"printOffset\" = 0.1905"
body "Solid1"
